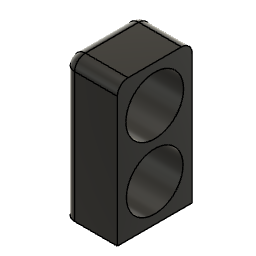
316592fce7f853e4 (Autodesk Fusion 360 archive; units mm, degrees)
design "センサーマウント小"
Autodesk Fusion 360 part; units mm, degrees
sketch "スケッチ1" plane through (0, 0, 0) normal (0, 1, 0) x (1, 0, 0)
  line L0 (0, 0) -> (5, 0)
  line L1 (5, 0) -> (5, 7)
  line L2 (5, 7) -> (0, 7)
  line L3 (0, 7) -> (0, 0)
  dimension "d1" = 5
  dimension "d2" = 7
  constraint horizontal L0
  constraint vertical L1
  constraint horizontal L2
  constraint vertical L3
  constraint coincident L0.start L3.end
  measures "d1" distance of L0.start L0.end
  measures "d2" distance of L0.start L2.end
extrude "押し出し4" add sketch "スケッチ1" along normal blind 13.15 and the other way blind 0
sketch "スケッチ2" plane through (0, 0, 0) normal (-1, 0, 0) x (0, 0, 1)
  line L0 (-7, 0) -> (0, 0)
  line L1 (0, 0) -> (0, 12)
  line L2 (0, 12) -> (-7, 12)
  line L3 (-7, 12) -> (-7, 0)
  line L4 (-12.7816, 6) -> (8, 6) construction
  line L5 (-13.4949, 12.65) -> (9, 12.65) construction
  line L6 (-13, 0.5) -> (9, 0.5) construction
  line L7 (-13.4949, 9.65) -> (9, 9.65) construction
  line L8 (-13, 3.5) -> (9, 3.5) construction
  line L9 (-3.5, -4.1964) -> (-3.5, 16) construction
  circle A0 centre (-3.5, 9.65) radius 2.7
  circle A1 centre (-3.5, 3.5) radius 2.65
  line L10 (-7, 0) -> (0, 0)
  dimension "d5" = 3
  dimension "d6" = 3
  dimension "d7" = 5.4
  dimension "d8" = 5.3
  dimension "d30" = 3.5
  dimension "d31" = 6.15
  constraint perpendicular L1 L4
  constraint perpendicular L3 L5
  constraint perpendicular L1 L6
  constraint perpendicular L5 L9
  constraint coincident L9 A0.centre
  constraint coincident L7 A0.centre
  constraint coincident L9 A1.centre
  constraint coincident L8 A1.centre
  measures "d7" diameter of A0
  measures "d8" diameter of A1
  measures "d30" distance of A1.centre L10
  measures "d31" distance of A0.centre A1.centre
extrude "押し出し5" cut sketch "スケッチ2" against normal blind 7 contours L2 A0 | L2 A0 | A1
sketch "スケッチ4" plane through (0, 0, 0) normal (0, -1, 0) x (1, 0, 0)
  line L0 (0, 0) -> (0, -7)
  line L1 (0, -7) -> (5, -7)
  line L2 (5, -7) -> (5, 0)
  line L3 (5, 0) -> (0, 0)
  circle A0 centre (5, -3.5) radius 2
  dimension "d19" = 4
  measures "d19" diameter of A0
fillet "フィレット1" radius 1 1 edges at (0, 13.15, -3.5)
fillet "フィレット2" radius 1 3 edges at (0, 6.075, -7) (0.2929, 12.8571, -7) (3, 13.15, -7)
fillet "フィレット3" radius 1 3 edges at (0, 6.075, 0) (0.2929, 12.8571, 0) (3, 13.15, 0)
equation "d15 = 12 mm + 1.15 mm"
equation "d31 = ( 5.4 / 2 ) * 1 mm + ( 5.3 / 2 ) * 1 mm + 0.8 mm"

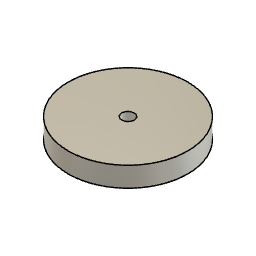
design "ホイール"
Autodesk Fusion 360 part; units mm, degrees
sketch "スケッチ1" plane through (0, 0, 0) normal (0, 1, 0) x (1, 0, 0)
  circle A0 centre (0, 0) radius 2.5
  circle A1 centre (0, 0) radius 24
  dimension "d1" = 5
  dimension "d2" = 48
  constraint coincident A0.centre A1.centre
  measures "d1" diameter of A0
  measures "d2" diameter of A1
extrude "押し出し1" add sketch "スケッチ1" along normal blind 8

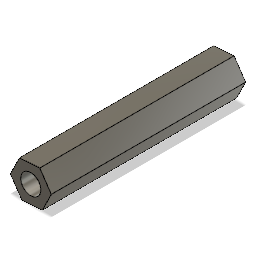
design "スペーサ"
Autodesk Fusion 360 part; units mm, degrees
sketch "スケッチ1" plane through (0, 0, 0) normal (0, 0, 1) x (1, 0, 0)
  line L0 (1.395, 2.8526) -> (-1.7729, 2.6344)
  line L1 (-1.7729, 2.6344) -> (-3.1679, -0.2182)
  line L2 (-3.1679, -0.2182) -> (-1.395, -2.8526)
  line L3 (-1.395, -2.8526) -> (1.7729, -2.6344)
  line L4 (1.7729, -2.6344) -> (3.1679, 0.2182)
  line L5 (3.1679, 0.2182) -> (1.395, 2.8526)
  circle A0 centre (0, 0) radius 1.55
  dimension "d1" = 2.75
  dimension "d4" = 3.1
  constraint coincident A0.centre origin
  measures "d1" distance of A0.centre L5
  measures "d4" diameter of A0
extrude "押し出し1" add sketch "スケッチ1" along normal blind 30
equation "d1 = ( 5.5 / 2 ) * 1 mm"

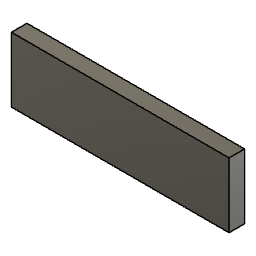
design "壁"
Autodesk Fusion 360 part; units mm, degrees
sketch "スケッチ1" plane through (0, 0, 0) normal (0, 1, 0) x (1, 0, 0)
  line L0 (0, 0) -> (168, 0)
  line L1 (168, 0) -> (168, 12)
  line L2 (168, 12) -> (0, 12)
  line L3 (0, 12) -> (0, 0)
  dimension "d1" = 168
  dimension "d2" = 12
  constraint horizontal L0
  constraint vertical L1
  constraint horizontal L2
  constraint vertical L3
  constraint coincident L0.start L3.end
  measures "d1" distance of L0.start L0.end
  measures "d2" distance of L0.start L2.end
extrude "押し出し1" add sketch "スケッチ1" along normal blind 50

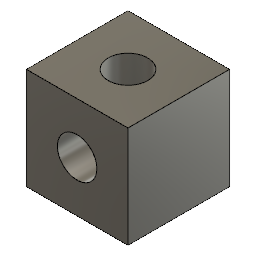
design "角型スペーサ"
Autodesk Fusion 360 part; units mm, degrees
sketch "スケッチ1" plane through (0, 0, 0) normal (0, 0, 1) x (1, 0, 0)
  line L0 (0, 0) -> (8, 0)
  line L1 (8, 0) -> (8, 8)
  line L2 (8, 8) -> (0, 8)
  line L3 (0, 8) -> (0, 0)
  circle A0 centre (4, 4) radius 1.55
  dimension "d1" = 8
  dimension "d4" = 3.1
  constraint horizontal L0
  constraint vertical L1
  constraint horizontal L2
  constraint vertical L3
  constraint coincident L0.start L3.end
  measures "d1" distance of L0.start L2.end
  measures "d4" diameter of A0
extrude "押し出し1" add sketch "スケッチ1" along normal blind 8
sketch "スケッチ2" plane through (0, 0, 0) normal (0, -1, 0) x (1, 0, 0)
  line L0 (0, 0) -> (8, 0)
  line L1 (8, 0) -> (8, 8)
  line L2 (8, 8) -> (0, 8)
  line L3 (0, 8) -> (0, 0)
  circle A0 centre (4, 4) radius 1.55
  dimension "d5" = 3.1
  measures "d5" diameter of A0
extrude "押し出し2" cut sketch "スケッチ2" against normal blind 9 contours A0

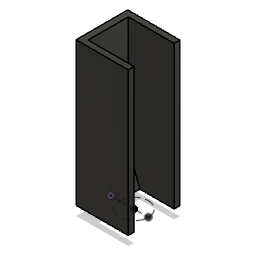
design "センサーマウント大"
Autodesk Fusion 360 part; units mm, degrees
sketch "スケッチ1" plane through (0, 0, 0) normal (0, 1, 0) x (1, 0, 0)
  line L0 (-6.5318, 0) -> (8, 0) construction
  line L1 (0, 7) -> (0, -8) construction
  line L2 (0, 0.55) -> (-1, 0.55)
  line L3 (0, -0.55) -> (-1, -0.55)
  line L4 (0, 0.55) -> (1, 0.55)
  line L5 (0, -0.55) -> (1, -0.55)
  arc A0 (-1, 0.55) -> (-1, -0.55) centre (-1, 0) ccw
  arc A1 (1, -0.55) -> (1, 0.55) centre (1, 0) ccw
  dimension "d5" = 0.55
  constraint horizontal L0
  constraint perpendicular L0 L1
  constraint coincident L1 L2.start
  constraint perpendicular L1 L2
  constraint symmetric L0 L2.start L3.start
  constraint symmetric L0 L2.end L3.end
  constraint symmetric L1 L2.start L4.start
  constraint symmetric L1 L2.end L4.end
  constraint symmetric L1 L3.start L5.start
  constraint symmetric L1 L3.end L5.end
  constraint tangent L3 A0
  constraint tangent L4 A1
  measures "d5" distance of L0 L2
extrude "押し出し1" add sketch "スケッチ1" against normal blind 1.6
sketch "スケッチ2" plane through (0, 0, 0) normal (0, 1, 0) x (1, 0, 0)
  line L0 (0, 0) -> (1.55, 0) construction
  line L1 (1.55, 0) -> (6.55, 0) construction
  circle A0 centre (4.05, 0) radius 2.5 construction
  dimension "d8" = 1.55
  dimension "d9" = 5
  constraint coincident L0.start origin
  constraint horizontal L0
  constraint parallel L0 L1
  constraint midpoint L1 A0.centre
  constraint coincident L0.end A0
  measures "d8" distance of L0.start L0.end
  measures "d9" distance of L0.end L1.end
sketch "スケッチ3" plane through (0, 0, 0) normal (0, 1, 0) x (1, 0, 0)
  line L0 (0, 0) -> (-1.55, 0) construction
  line L1 (-1.55, 0) -> (-1.55, 4.5)
  line L2 (-1.55, 4.5) -> (7.55, 4.5)
  line L3 (7.55, 4.5) -> (7.55, 0)
  line L4 (-1.55, 0) -> (-1.55, -4.5)
  line L5 (-1.55, -4.5) -> (7.55, -4.5)
  line L6 (7.55, -4.5) -> (7.55, 0)
  dimension "d10" = 1.55
  dimension "d11" = 4.5
  dimension "d12" = 9.1
  constraint coincident L0.start origin
  constraint horizontal L0
  constraint vertical L1
  constraint perpendicular L1 L2
  constraint perpendicular L2 L3
  constraint symmetric L1.start L0 L4.start
  constraint symmetric L0 L1.end L4.end
  constraint symmetric L0 L2.end L5.end
  constraint symmetric L0 L3.end L6.end
  measures "d10" distance of L0.start L0.end
  measures "d11" distance of L0.end L1.end
  measures "d12" distance of L1.end L2.end
extrude "押し出し2" add sketch "スケッチ3" along normal blind 25
sketch "スケッチ4" plane through (7.55, 0, 0) normal (1, 0, 0) x (0, 0, -1)
  line L0 (-4.5, 0) -> (4.5, 0)
  line L1 (4.5, 0) -> (4.5, 25)
  line L2 (4.5, 25) -> (-4.5, 25)
  line L3 (-4.5, 25) -> (-4.5, 0)
  line L4 (0, 16.5) -> (0, -2.5) construction
  line L5 (-3.8767, 7.5) -> (4, 7.5) construction
  line L6 (0, 25) -> (-3.5, 25)
  line L7 (-3.5, 25) -> (-3.5, 0)
  line L8 (-3.5, 0) -> (0, 0)
  line L9 (3.5, 0) -> (0, 0)
  line L10 (3.5, 25) -> (3.5, 0)
  line L11 (0, 25) -> (3.5, 25)
  dimension "d15" = 3.5
  constraint perpendicular L2 L4
  constraint perpendicular L1 L5
  constraint midpoint L2 L6.start
  constraint perpendicular L4 L6
  constraint coincident L0 L7.end
  constraint perpendicular L0 L7
  constraint coincident L8.end L9.end
  constraint symmetric L4 L6.start L11.start
  constraint symmetric L4 L6.end L10.start
  constraint symmetric L4 L7.end L9.start
  constraint symmetric L4 L8.end L9.end
  measures "d15" distance of L6.start L6.end
extrude "押し出し3" cut sketch "スケッチ4" against normal blind 6 contours L0 L2 L6 L7 L8 L9 L10 L11
sketch "スケッチ5" plane through (1.55, 0, 0) normal (1, 0, 0) x (0, 0, -1)
  line L0 (-3.5, 25) -> (3.5, 25)
  line L1 (3.5, 25) -> (3.5, 5)
  line L2 (3.5, 5) -> (-3.5, 5)
  line L3 (-3.5, 5) -> (-3.5, 25)
  dimension "d19" = 7
  dimension "d20" = 20
  constraint horizontal L0
  constraint vertical L1
  constraint horizontal L2
  constraint vertical L3
  measures "d19" distance of L0.start L0.end
  measures "d20" distance of L0.start L2.end
extrude "押し出し4" cut sketch "スケッチ5" against normal blind 2
draft "勾配1" angle -20 neutral plane through (0, 0, 0) pull (0, -1, 0) 1 faces at (1.55, 3.3333, 0)
equation "d8 = 1 mm + 0.55 mm"
equation "d10 = 1 mm + 0.55 mm"
equation "d12 = 3.1 mm + 6.0 mm"

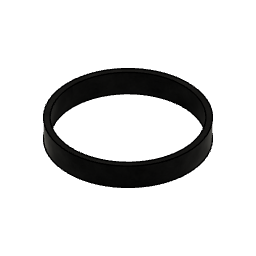
design "タイヤ"
Autodesk Fusion 360 part; units mm, degrees
sketch "スケッチ1" plane through (0, 0, 0) normal (0, 1, 0) x (1, 0, 0)
  circle A0 centre (0, 0) radius 24
  circle A1 centre (0, 0) radius 26
  dimension "d1" = 48
  dimension "d2" = 52
  constraint coincident A0.centre A1.centre
  measures "d1" diameter of A0
  measures "d2" diameter of A1
extrude "押し出し1" add sketch "スケッチ1" along normal blind 8
equation "d2 = 48 mm + 4 mm"

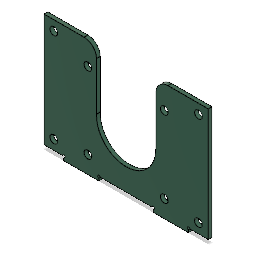
design "モーターマウント"
Autodesk Fusion 360 part; units mm, degrees
sketch "スケッチ1" plane through (0, 0, 0) normal (0, 0, 1) x (1, 0, 0)
  line L0 (25.35, -22.6) -> (25.35, -21)
  line L1 (-11.9915, -0.4526) -> (-11.9915, 20)
  line L2 (12, 0) -> (12, 20)
  arc A0 (-11.9915, 0.4526) -> (8.9572, -7.9855) centre (0, 0) ccw
  arc A1 (8.9572, -7.9855) -> (12, 0) centre (0, 0) ccw
  line L3 (11, -21) -> (-11, -21)
  line L4 (-11, -21) -> (-11, -22.6)
  line L5 (11, -22.6) -> (11, -21)
  line L6 (-25.35, -22.6) -> (-11, -22.6)
  line L7 (11, -22.6) -> (25.35, -22.6)
  line L8 (15.5, 15.5) -> (-15.5, -15.5) construction
  line L9 (-15.5, 15.5) -> (15.5, -15.5) construction
  circle A2 centre (-15.5, 15.5) radius 1.55
  circle A3 centre (-15.5, -15.5) radius 1.55
  circle A4 centre (15.5, -15.5) radius 1.55
  circle A5 centre (15.5, 15.5) radius 1.55
  line L10 (-33.35, 25) -> (-33.35, -21)
  line L11 (-33.35, -21) -> (-25.35, -21)
  line L12 (33.35, 25) -> (33.35, -21)
  line L13 (33.35, -21) -> (25.35, -21)
  line L14 (-33.35, 25) -> (-16.9915, 25)
  line L15 (17, 25) -> (33.35, 25)
  line L16 (-25.35, -21) -> (-25.35, -22.6)
  circle A6 centre (-25.35, -21) radius 0.5
  circle A7 centre (-11, -21) radius 0.5
  circle A8 centre (11, -21) radius 0.5
  circle A9 centre (25.35, -21) radius 0.5
  line L17 (-33.35, 25) -> (-25.35, 25)
  line L18 (-25.35, 25) -> (-25.35, 17)
  line L19 (-33.35, 17) -> (-33.35, 25)
  line L20 (-33.35, -21) -> (-25.35, -21)
  line L21 (-25.35, -21) -> (-25.35, -13)
  line L22 (-33.35, -13) -> (-33.35, -21)
  line L23 (33.35, 25) -> (25.35, 25)
  line L24 (25.35, 25) -> (25.35, 17)
  line L25 (33.35, 17) -> (33.35, 25)
  line L26 (33.35, -21) -> (25.35, -21)
  line L27 (25.35, -21) -> (25.35, -13)
  line L28 (33.35, -13) -> (33.35, -21)
  line L29 (0, 11) -> (0, -6)
  line L30 (-60, 0) -> (-22.7376, 0)
  circle A10 centre (-29.35, 21) radius 1.55
  circle A11 centre (29.35, 21) radius 1.55
  circle A12 centre (-29.35, -17.0232) radius 1.55
  circle A13 centre (29.35, -17.0232) radius 1.55
  arc A14 (-11.9915, 20) -> (-16.9915, 25) centre (-16.9915, 20) ccw
  arc A15 (17, 25) -> (12, 20) centre (17, 20) ccw
  point P0 (82.8077, 25)
  dimension "d5" = 24
  dimension "d11" = 31
  dimension "d12" = 31
  dimension "d13" = 3.1
  dimension "d14" = 3.1
  dimension "d15" = 3.1
  dimension "d16" = 3.1
  dimension "d25" = 14.35
  dimension "d43" = 11
  dimension "d44" = 11
  dimension "d45" = 22.6
  dimension "d46" = 21
  dimension "d49" = 22.6
  dimension "d51" = 33.35
  dimension "d52" = 33.35
  dimension "d53" = 1
  dimension "d54" = 1
  dimension "d55" = 1
  dimension "d56" = 1
  dimension "d57" = 8
  dimension "d58" = 8
  dimension "d59" = 8
  dimension "d60" = 8
  dimension "d61" = 8
  dimension "d62" = 8
  dimension "d63" = 8
  dimension "d64" = 8
  dimension "d83" = 3.1
  dimension "d84" = 3.1
  dimension "d85" = 3.1
  dimension "d86" = 3.1
  dimension "d87" = 14.35
  dimension "d88" = 5
  dimension "d89" = 5
  constraint coincident A0.centre A1.centre
  constraint coincident L1.start A0
  constraint tangent L2 A0
  constraint coincident L1 A0.start
  constraint concentric A0 A1
  constraint perpendicular L3 L4
  constraint parallel L4 L5
  constraint horizontal L3
  constraint coincident L8 A0.centre
  constraint coincident L9 A0.centre
  constraint coincident L9.start A2.centre
  constraint coincident L8.end A3.centre
  constraint coincident L9.end A4.centre
  constraint coincident L8.start A5.centre
  constraint perpendicular L3 L10
  constraint collinear L14 L15
  constraint perpendicular L6 L16
  constraint coincident L11.end L16.start
  constraint coincident L3.end L4.start
  constraint coincident L3.start L5.end
  constraint coincident L0.end L13.end
  constraint horizontal L17
  constraint vertical L18
  constraint vertical L19
  constraint horizontal L20
  constraint vertical L21
  constraint vertical L22
  constraint horizontal L23
  constraint vertical L24
  constraint vertical L25
  constraint horizontal L26
  constraint vertical L27
  constraint vertical L28
  constraint vertical L29
  constraint horizontal L30
  constraint tangent L14 A14
  constraint tangent L1 A14
  constraint tangent L15 A15
  constraint tangent L2 A15
  measures "d5" diameter of A0
  measures "d11" distance of L8.end L9.end
  measures "d12" distance of L9.start L8.end
  measures "d13" diameter of A2
  measures "d14" diameter of A3
  measures "d15" diameter of A4
  measures "d16" diameter of A5
  measures "d25" distance of L0 L5
  measures "d43" distance of A0.centre L4
  measures "d44" distance of L5 A0.centre
  measures "d45" distance of A0.centre L6
  measures "d46" distance of A0.centre L3
  measures "d49" distance of A0.centre L7
  measures "d51" distance of A0.centre L10
  measures "d52" distance of A0.centre L12
  measures "d53" diameter of A6
  measures "d54" diameter of A7
  measures "d55" diameter of A8
  measures "d56" diameter of A9
  measures "d57" distance of L10.start L17.end
  measures "d58" distance of L10.start L19.start
  measures "d59" distance of L10.end L11.end
  measures "d60" distance of L10.end L22.start
  measures "d61" distance of L12.start L23.end
  measures "d62" distance of L12.start L25.start
  measures "d63" distance of L12.end L0.end
  measures "d64" distance of L12.end L28.start
  measures "d83" diameter of A10
  measures "d84" diameter of A11
  measures "d85" diameter of A12
  measures "d86" diameter of A13
  measures "d87" distance of L6.start L4
  measures "d88" radius of A14
  measures "d89" radius of A15
extrude "押し出し1" add sketch "スケッチ1" along normal blind 1.57 contours L0 L1 L2 A0 A1 L3 L4 L5 L6 L7 L10 L11 L12 L13 L14 L15 L16 A6 A7 A8 A9 L17 L19 L20 L22 L23 L25 L26 L28 A14 A15 sketch seen with x (1, 0, 0) y (0, 1, 0) z (0, 0, 1) at (33.35, 22.6, 0) in component "ボード"
component "ボード" placed x (1, 0, 0) y (0, 1, 0) z (0, 0, 1) at (-33.35, -22.6, 0)
equation "d45 = 21 mm + 1.6 mm"
equation "d51 = ( 50.7 / 2 + 8 ) * 1 mm"
equation "d52 = ( 50.7 / 2 + 8 ) * 1 mm"
named bodies: "ボード"
